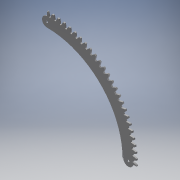
# Autodesk Inventor part: Spur_Outer_10-1
Saved by Autodesk Inventor 2019 (Build 230136000, 136)
## iProperties
Created: 2019-05-31
Part Number: Spur_Outer_10-1
Material: Steel
Document SubType Name: Modeling
Designer: Jorian Brusind
Categories: <?xml version="1.0" encoding="UTF-16"?> <MemberInstance><Categories><FamilyTemplate><FamilyTemplateParameter ValueType="xs:double" Id="1" ObjectReferenceKey="da_z" ObjectType="kUserParameterObject"/><FamilyTemplateParameter ValueType="xs:double" Id="2" ObjectReferenceKey="da_b" ObjectType="kUserParameterObject"/><FamilyTemplateParameter ValueType="xs:double" Id="3" ObjectReferenceKey="da_beta" ObjectType="kUserParameterObject"/><FamilyTemplateParameter ValueType="xs:double" Id="4" ObjectReferenceKey="da_da" ObjectType="kUserParameterObject"/><FamilyTemplateParameter ValueType="xs:double" Id="5" ObjectReferenceKey="da_aw" ObjectType="kUserParameterObject"/><FamilyTemplateParameter ValueType="xs:string" Id="6" ObjectReferenceKey="EAIAABAAAACIAQAAAAAAAIAAAAAAAAAA" ObjectType="83910656" SubObjectId="SurfaceGeometry"/></FamilyTemplate><ParamToTemplateMap><ParamToTemplate CategoryParameter="//CategoryParameter[@InternalName='046C89C9-8512-4d59-83FE-43B91F4F132A']" TemplateParameter="1"/><ParamToTemplate CategoryParameter="//CategoryParameter[@InternalName='2552DF32-E462-4b46-AEBF-C6C7768E72AC']" TemplateParameter="2"/><ParamToTemplate CategoryParameter="//CategoryParameter[@InternalName='C9EE641D-15FC-4fae-A226-E94C4372FDD7']" TemplateParameter="3"/><ParamToTemplate><ParamToTemplate CategoryParameter="//CategoryParameter[@InternalName='00B6519A-459B-49c7-AD84-2E56D39A5744']" ConstantValue="0.348307"/></ParamToTemplate><ParamToTemplate><ParamToTemplate CategoryParameter="//CategoryParameter[@InternalName='04B31F0E-C7A6-4894-AA32-9629BEFACF47']" ConstantValue="1.000000"/></ParamToTemplate><ParamToTemplate><ParamToTemplate CategoryParameter="//CategoryParameter[@InternalName='43CBEC2E-7847-49e7-A936-2F7889FCB2D9']" ConstantValue="0.250000"/></ParamToTemplate><ParamToTemplate><ParamToTemplate CategoryParameter="//CategoryParameter[@InternalName='B1EFC894-105D-4ebd-86BF-FA20ED196853']" ConstantValue="0.350000"/></ParamToTemplate><ParamToTemplate><ParamToTemplate CategoryParameter="//CategoryParameter[@InternalName='51175063-3D10-4879-93E8-6246FE8B403D']" ConstantValue="2060000000.000000"/></ParamToTemplate><ParamToTemplate><ParamToTemplate CategoryParameter="//CategoryParameter[@InternalName='A3A52E27-4454-46a9-B0BD-C932399B70AF']" ConstantValue="0.300000"/></ParamToTemplate><ParamToTemplate><ParamToTemplate CategoryParameter="//CategoryParameter[@InternalName='91B76062-C214-41d9-B1B9-14D2AB99603D']" ConstantValue="0.300000"/></ParamToTemplate><ParamToTemplate><ParamToTemplate CategoryParameter="//CategoryParameter[@InternalName='374E806E-8B8A-4dda-A9AA-1039D6500AD2']" ConstantValue="3.333333"/></ParamToTemplate><ParamToTemplate><ParamToTemplate CategoryParameter="//CategoryParameter[@InternalName='2D373A89-B862-43d6-8D0B-0CBF12AB9F6C']" ConstantValue="0.523599"/></ParamToTemplate><ParamToTemplate CategoryParameter="//CategoryParameter[@InternalName='37777632-D6A2-4fac-9D53-DB8ACD95C989']" TemplateParameter="4"/><ParamToTemplate CategoryParameter="//CategoryParameter[@InternalName='FD1017F1-B727-4f7e-9707-0F86F1FF9423']" TemplateParameter="5"/><ParamToTemplate><ParamToTemplate CategoryParameter="//CategoryParameter[@InternalName='9E1B4470-B2D3-4ff1-B813-535BB4CDF51A']" ConstantValue="3520000.000000"/></ParamToTemplate><ParamToTemplate><ParamToTemplate CategoryParameter="//CategoryParameter[@InternalName='F8452263-BFF6-458c-9FB1-07C4B99E95CD']" ConstantValue="11400000.000000"/></ParamToTemplate><ParamToTemplate><ParamToTemplate CategoryParameter="//CategoryParameter[@InternalName='3E3BB259-FD49-497f-8171-6EBC954A3479']" ConstantValue="2.000000"/></ParamToTemplate><ParamToTemplate CategoryParameter="//CategoryParameter[@InternalName='27C3BAF2-7550-4e4b-AE2C-0DB134B7D9B7']" TemplateParameter="6"/></ParamToTemplateMap><Category DisplayName="Gear" InternalName="DC85795E-93AB-48d5-8EEE-5A27447B64BD" Mnemonic="Gear"><CategoryParameter DisplayName="z" InternalName="046C89C9-8512-4d59-83FE-43B91F4F132A" Mnemonic="z"/><CategoryParameter DisplayName="b" InternalName="2552DF32-E462-4b46-AEBF-C6C7768E72AC" Mnemonic="b"/><CategoryParameter DisplayName="||b|" InternalName="C9EE641D-15FC-4fae-A226-E94C4372FDD7" Mnemonic="beta"/><CategoryParameter DisplayName="x" InternalName="00B6519A-459B-49c7-AD84-2E56D39A5744" Mnemonic="x"/><CategoryParameter DisplayName="a*" InternalName="04B31F0E-C7A6-4894-AA32-9629BEFACF47" Mnemonic="a"/><CategoryParameter DisplayName="c*" InternalName="43CBEC2E-7847-49e7-A936-2F7889FCB2D9" Mnemonic="c"/><CategoryParameter DisplayName="r|.f|*" InternalName="B1EFC894-105D-4ebd-86BF-FA20ED196853" Mnemonic="rf"/><CategoryParameter DisplayName="E" InternalName="51175063-3D10-4879-93E8-6246FE8B403D" Mnemonic="E"/><CategoryParameter DisplayName="||m|" InternalName="A3A52E27-4454-46a9-B0BD-C932399B70AF" Mnemonic="mi"/><Category DisplayName="SpurGear" InternalName="26C5A22E-A91E-4dfd-A3B3-23CCAFAE1764" Mnemonic="SpurGear"><CategoryParameter DisplayName="m" InternalName="91B76062-C214-41d9-B1B9-14D2AB99603D" Mnemonic="m"/><CategoryParameter DisplayName="P" InternalName="374E806E-8B8A-4dda-A9AA-1039D6500AD2" Mnemonic="PP"/><CategoryParameter DisplayName="||a|" InternalName="2D373A89-B862-43d6-8D0B-0CBF12AB9F6C" Mnemonic="alpha"/><CategoryParameter DisplayName="d|.a|" InternalName="37777632-D6A2-4fac-9D53-DB8ACD95C989" Mnemonic="da"/><CategoryParameter DisplayName="a|.w|" InternalName="FD1017F1-B727-4f7e-9707-0F86F1FF9423" Mnemonic="aw"/><CategoryParameter DisplayName="||s||.Flim|" InternalName="9E1B4470-B2D3-4ff1-B813-535BB4CDF51A" Mnemonic="sFlim"/><CategoryParameter DisplayName="||s||.Hlim|" InternalName="F8452263-BFF6-458c-9FB1-07C4B99E95CD" Mnemonic="sHlim"/><CategoryParameter DisplayName="type" InternalName="3E3BB259-FD49-497f-8171-6EBC954A3479" Mnemonic="type"/><CategoryParameter DisplayName="PitchDiameter" InternalName="27C3BAF2-7550-4e4b-AE2C-0DB134B7D9B7" Mnemonic="IDS_PITCHDIAM"/></Category></Category></Categories></MemberInstance>
Density: 1 g/cm^3
Appearance: Steel
CustomPartVersion: 1
Author: Jorian Brusind
Autodesk Inventor part; units mm, degrees
sketch "Sketch1" plane through (0, 0, 0) normal (0, 0, 1) x (1, 0, 0)
  circle A0 centre (0, 0) radius 154.0352
  dimension "d0" = 308.0704
  constraints: 1 centre point
  measures "d0" diameter of A0
extrude "Extrusion1" add sketch "Sketch1" along normal blind 2.5
ref_plane "Work Plane2" through (0, 0, 1.25) normal (0, 0, 1) x (1, 0, 0)
sketch "Sketch2" plane through (0, 0, 0) normal (0, 0, -1) x (-1, 0, 0)
  circle A0 centre (0, 0) radius 154.0352 projected
  circle A1 centre (0, 0) radius 150.9497
  dimension "d3" = 301.8995
  constraints: 1 centre point, 1 coincident
  measures "d3" diameter of A1
surface extrude "Pitch Diameter" sketch "Sketch2" against normal through all shown no curves A1
ref_plane "Work Plane8" through (0, 0, 0) normal (0.9995066, 0.0314108, 0) x (0, 0, 1)
ref_plane "Work Plane9" through (0, 0, 0) normal (1, 0, 0) x (0, 1, 0)
spur gear teeth "Spur Gear" teeth 100 pitch diameter 300 tip diameter 308.0704 root diameter 294.5898 face width 2.5 start plane through (0, 0, 0) normal (0, 0, -1) x (-1, 0, 0)
sketch "Sketch5" plane through (0, 0, 2.5) normal (0, 0, 1) x (1, 0, 0)
  arc A0 (0, 154.035) -> (154.035, 0) centre (0, 0) ccw
  line L0 (0, 0) -> (0, 154.035) construction
  line L1 (0, 0) -> (154.035, 0) construction
  line L2 (0, 0) -> (154.035, 0) construction
  arc A1 (1.2098, 154.0305) -> (-1.2098, 154.0305) centre (0, 0) ccw projected
  line L3 (0, 154.035) -> (0, 0)
  line L4 (0, 0) -> (154.035, 0)
  dimension "d55" = 154.035
  dimension "d56" = 90
  dimension "d57" = 90
  constraints: 10 end point, 2 horizontal, 2 point on circle, 1 centre point, 1 coincident, 1 collinear, 1 perpendicular
  measures "d55" radius of A0
  measures "d56" angle of L1 L0
  measures "d57" angle of L2 L0
extrude "Extrusion3" cut sketch "Sketch5" against normal blind 20 fills toward (-0.05, 77.0175) open curves L3 L4
sketch "Sketch6" plane through (0, 0, 2.5) normal (0, 0, 1) x (1, 0, 0)
  line L0 (0, 0) -> (0, 154.0352) projected
  line L1 (0, 0) -> (154.0352, 0) projected
  arc A0 (130, 0) -> (0, 130) centre (0, 0) ccw
  line L2 (0, 130) -> (0, 0)
  line L3 (0, 0) -> (130, 0)
  dimension "d61" = 130
  constraints: 4 end point, 2 collinear, 2 point on circle, 1 centre point, 1 coincident, 1 point on line
  measures "d61" radius of A0
extrude "Extrusion4" cut sketch "Sketch6" against normal blind 20
sketch "Sketch7" plane through (0, 0, 2.5) normal (0, 0, 1) x (1, 0, 0)
  line L0 (0, 154.0352) -> (0, 130) projected
  line L1 (0, 130) -> (0, 138.5)
  circle A0 centre (0, 138.5) radius 8.5
  arc A1 (130, 0) -> (0, 130) centre (0, 0) ccw projected
  line L2 (130, 0) -> (138.5, 0)
  line L3 (154.0352, 0) -> (130, 0) projected
  circle A2 centre (138.5, 0) radius 8.5
  dimension "d64" = 8.5
  dimension "d65" = 17
  dimension "d66" = 8.5
  dimension "d67" = 17
  constraints: 4 end point, 2 centre point, 2 coincident, 2 point on line
  measures "d64" distance of L0.end L1.end
  measures "d65" diameter of A0
  measures "d66" distance of L2.start L2.end
  measures "d67" diameter of A2
extrude "Extrusion5" add sketch "Sketch7" against normal blind 1.25 contours L0 A0 | L0 A0
sketch "Sketch8" plane through (0, 0, 2.5) normal (0, 0, 1) x (1, 0, 0)
  arc A0 (130, 0) -> (0, 130) centre (0, 0) ccw projected
  line L0 (130, 0) -> (138.5, 0)
  line L1 (154.0352, 0) -> (130, 0) projected
  circle A1 centre (138.5, 0) radius 8.5
  dimension "d70" = 8.5
  dimension "d71" = 17
  constraints: 2 end point, 1 centre point, 1 coincident, 1 point on line
  measures "d70" distance of L0.start L0.end
  measures "d71" diameter of A1
extrude "Extrusion6" cut sketch "Sketch8" against normal blind 1.25
sketch "Sketch9" plane through (0, 0, 0) normal (0, 0, -1) x (-1, 0, 0)
  line L0 (-147, 0) -> (-130, 0) projected
  line L1 (-130, 0) -> (-138.5, 0)
  line L2 (-130, 0) -> (-121.5, 0) construction
  circle A0 centre (-138.5, 0) radius 8.5
  point P0 (0, 0)
  dimension "d74" = 8.5
  dimension "d75" = 180
  dimension "d76" = 17
  constraints: 4 end point, 2 collinear, 1 centre point, 1 coincident, 1 horizontal
  measures "d74" distance of L0.end L1.end
  measures "d75" angle of L1 L2
  measures "d76" diameter of A0
extrude "Extrusion7" add sketch "Sketch9" against normal blind 1.25
sketch "Sketch10" plane through (0, 0, 0) normal (0, 0, -1) x (-1, 0, 0)
  line L0 (0, 130) -> (0, 154.0352) projected
  line L1 (0, 130) -> (0, 138.5)
  arc A0 (0, 130) -> (0, 147) centre (0, 138.5) ccw projected
  circle A1 centre (0, 138.5) radius 8.5
  point P0 (0, 0)
  dimension "d79" = 8.5
  constraints: 2 end point, 1 coincident, 1 point on line, 1 vertical alignment, 2 other
  measures "d79" distance of L0.start L1.end
extrude "Extrusion8" cut sketch "Sketch10" against normal blind 1.25
sketch "Sketch11" plane through (0, 0, 0) normal (0, 0, -1) x (-1, 0, 0)
  arc A0 (-147, 0) -> (-130, 0) centre (-138.5, 0) ccw projected
  circle A1 centre (-138.5, 0) radius 1.75
  arc A2 (0, 147) -> (0, 130) centre (0, 138.5) ccw projected
  circle A3 centre (0, 138.5) radius 1.75
  point P0 (0, 0)
  dimension "d82" = 3.5
  dimension "d83" = 3.5
  constraints: 2 centre point, 2 coincident
  measures "d82" diameter of A1
  measures "d83" diameter of A3
extrude "Extrusion9" cut sketch "Sketch11" against normal blind 2.5
equation "\"d0\" = da_da"
equation "\"d1\" = da_b"
equation "\"d3\" = da_dw"
equation "\"d16\" = da_aw"
equation "\"d43\" = da_aw"
equation "\"d46\" = da_aw"
equation "\"da_da\" = 308.070424"
equation "\"da_b\" = 2.5"
equation "\"da_dw\" = 301.899472"
equation "\"da_aw\" = 164.535212"
body "Solid1"
body "Srf1"
